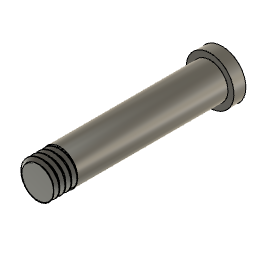
Axle wheel front v0 (Autodesk Fusion 360 design; units mm, degrees)
Autodesk Fusion 360 part; units mm, degrees
mesh "Mesh1" [no effect] in component "axle wheel front 2 "
sketch "axle wheel front" plane through (0, 0, 0) normal (0, 0, 1) x (1, 0, 0) in component "axle wheel front 2 "
  circle A0 centre (0.0009, 0.0001) radius 3.9999
  circle A1 centre (0.0009, 0.0001) radius 2.9983
  constraint concentric A0 A1
extrude "Extrude1" add sketch "axle wheel front" along normal blind 2 contours A0 | A1 makes body 1 in component "axle wheel front 2 "
extrude "Extrude2" add sketch "axle wheel front" along normal blind 27.2 contours A1 bodies 1 in component "axle wheel front 2 "
extrude "Extrude3" add 1 faces at (0.896, -1.0938, 27.2) along direction (0, 0, 1) blind 4 separate body on bodies 1 makes body 2 in component "axle wheel front 2 "
thread "Thread1" "ISO Metric profile 6.0 M6x1 6g" major diameter 5.884 minor diameter 4.7435 pitch 1 angle 60 modelled right hand crest width 0.1444 on face at (2.9843, -0.2985, 28.5333) crest through (2.9429, 0.0001, 26.95) on bodies 2 in component "axle wheel front 2 "
combine "Combine1" operation add target body 1 tool bodies 2 in component "axle wheel front 2 "
component "axle wheel front 2 " placed x (0, 0, -1) y (1, 0, 0) z (0, -1, 0) at (72.0301, 41.3349, 5.5736)
component "axle wheel front 1" placed x (0, 1, 0) y (-1, 0, 0) z (0, 0, 1) at (-0.3027, -4.2307, -70.0813) in component "axle wheel front 2 "
component "axle wheel front 2" placed x (0, 1, 0) y (-1, 0, 0) z (0, 0, 1) at (-0.3027, -4.2307, -70.0813) in component "axle wheel front 2 "
named bodies: "axle wheel front"
